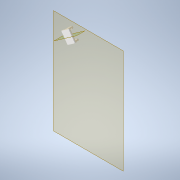
# Autodesk Inventor part: Omniscope_Camera_fix
Saved by Autodesk Inventor 2022 (Build 260153000, 153)
## iProperties
Created: 2022-05-26
Part Number: Omniscope_Camera_fix
Material: Generisch
Document SubType Name: Modeling
Designer: diederichbenedict
Density: 1 g/cm^3
Appearance: Vorgabe
Author: diederichbenedict
Autodesk Inventor part; units mm, degrees
ref_plane "YZ Plane" through (0, 0, 0) normal (1, 0, 0) x (0, 1, 0)
ref_plane "XZ Plane" through (0, 0, 0) normal (0, 1, 0) x (-1, 0, 0)
ref_plane "XY Plane" through (0, 0, 0) normal (0, 0, 1) x (1, 0, 0)
ref_plane "Arbeitsebene1" through (8.2312, -3.2392, 2) normal (0, 0, 1) x (1, 0, 0)
sketch "Skizze1" plane through (8.2312, -3.2392, 2) normal (0, 0, 1) x (1, 0, 0)
  arc A0 (-29.666, 52.3362) -> (-30.2278, 49.15) centre (-26.4114, 50.1197) ccw projected
  line L0 (-30.4697, 49.0886) -> (-31.8651, 51.0813) projected
  line L1 (-27.3731, 44.6661) -> (-28.7684, 46.6589) projected
  line L2 (-25.3803, 46.0614) -> (-27.3731, 44.6661) projected
  spline S0 degree 3 poles (-25.3803, 46.0614) (-25.4758, 46.0372) (-25.5717, 46.0164) (-25.765, 45.9815) (-25.8623, 45.9675) (-25.9823, 45.9545) (-26.0046, 45.9522) (-26.0633, 45.9468) (-26.0993, 45.944) (-26.1701, 45.9393) (-26.2048, 45.9374) (-26.2421, 45.9359) (-26.244, 45.9358) (-26.3578, 45.9313) (-26.4696, 45.9314) (-26.6928, 45.9405) (-26.8042, 45.9495) (-26.9899, 45.972) (-27.0643, 45.983) (-27.2355, 46.0132) (-27.3315, 46.0336) (-27.5218, 46.0812) (-27.6161, 46.1083) (-27.7358, 46.1473) (-27.7619, 46.1561) (-27.8204, 46.1765) (-27.8532, 46.1884) (-27.9183, 46.2129) (-27.9507, 46.2255) (-27.9876, 46.2405) (-27.9928, 46.2426) (-28.0892, 46.282) (-28.1788, 46.3225) (-28.3547, 46.4094) (-28.4411, 46.456) (-28.6083, 46.5538) (-28.6891, 46.6048) (-28.7684, 46.6589) knots 0 0 0 0 0.084049 0.084049 0.16831 0.16831 0.1875 0.1875 0.21875 0.21875 0.248427 0.248427 0.25 0.25 0.343462 0.343462 0.437098 0.437098 0.5 0.5 0.582124 0.582124 0.664424 0.664424 0.6875 0.6875 0.716281 0.716281 0.74522 0.74522 0.75 0.75 0.834095 0.834095 0.918237 0.918237 1 1 1 1 projected
  line L3 (-20.9578, 49.1581) -> (-22.9506, 47.7627) projected
  line L4 (-22.3532, 51.1509) -> (-20.9578, 49.1581) projected
  spline S1 degree 3 poles (-22.3532, 51.1509) (-22.3289, 51.0554) (-22.3081, 50.9594) (-22.2732, 50.7662) (-22.2592, 50.6689) (-22.2462, 50.5488) (-22.244, 50.5265) (-22.2385, 50.4679) (-22.2357, 50.4318) (-22.231, 50.3611) (-22.2292, 50.3263) (-22.2276, 50.289) (-22.2276, 50.2871) (-22.2231, 50.1733) (-22.2231, 50.0616) (-22.2322, 49.8384) (-22.2412, 49.727) (-22.2637, 49.5413) (-22.2747, 49.4668) (-22.3049, 49.2957) (-22.3254, 49.1997) (-22.3729, 49.0094) (-22.4, 48.915) (-22.4391, 48.7954) (-22.4479, 48.7693) (-22.4682, 48.7107) (-22.4801, 48.678) (-22.5046, 48.6128) (-22.5173, 48.5804) (-22.5322, 48.5436) (-22.5343, 48.5384) (-22.5738, 48.442) (-22.6142, 48.3524) (-22.7012, 48.1764) (-22.7477, 48.09) (-22.8455, 47.9229) (-22.8966, 47.842) (-22.9506, 47.7627) knots 0 0 0 0 0.084049 0.084049 0.16831 0.16831 0.1875 0.1875 0.21875 0.21875 0.248427 0.248427 0.25 0.25 0.343462 0.343462 0.437098 0.437098 0.5 0.5 0.582124 0.582124 0.664424 0.664424 0.6875 0.6875 0.716281 0.716281 0.74522 0.74522 0.75 0.75 0.834095 0.834095 0.918237 0.918237 1 1 1 1 projected
  line L5 (-25.4498, 55.5734) -> (-24.0545, 53.5806) projected
  line L6 (-27.4426, 54.178) -> (-25.4498, 55.5734) projected
  spline S2 degree 3 poles (-27.4426, 54.178) (-27.3471, 54.2023) (-27.2511, 54.2231) (-27.0579, 54.2579) (-26.9606, 54.272) (-26.8406, 54.285) (-26.8183, 54.2872) (-26.7596, 54.2926) (-26.7236, 54.2955) (-26.6528, 54.3001) (-26.6181, 54.302) (-26.5807, 54.3035) (-26.5789, 54.3036) (-26.4651, 54.3081) (-26.3533, 54.308) (-26.1301, 54.299) (-26.0187, 54.29) (-25.833, 54.2675) (-25.7586, 54.2564) (-25.5874, 54.2262) (-25.4914, 54.2058) (-25.3011, 54.1582) (-25.2067, 54.1311) (-25.0871, 54.0921) (-25.061, 54.0833) (-25.0025, 54.0629) (-24.9697, 54.0511) (-24.9046, 54.0266) (-24.8722, 54.0139) (-24.8353, 53.999) (-24.8301, 53.9969) (-24.7337, 53.9574) (-24.6441, 53.917) (-24.4681, 53.83) (-24.3817, 53.7835) (-24.2146, 53.6857) (-24.1337, 53.6346) (-24.0545, 53.5806) knots 0 0 0 0 0.084049 0.084049 0.16831 0.16831 0.1875 0.1875 0.21875 0.21875 0.248427 0.248427 0.25 0.25 0.343462 0.343462 0.437098 0.437098 0.5 0.5 0.582124 0.582124 0.664424 0.664424 0.6875 0.6875 0.716281 0.716281 0.74522 0.74522 0.75 0.75 0.834095 0.834095 0.918237 0.918237 1 1 1 1 projected
  line L7 (-27.0245, 40.5346) -> (-35.6282, 52.8219)
  line L8 (-35.6282, 52.8219) -> (-25.7984, 59.7048)
  line L9 (-25.7984, 59.7048) -> (-17.1947, 47.4175)
  line L10 (-17.1947, 47.4175) -> (-27.0245, 40.5346)
  line L11 (-27.0245, 40.5346) -> (-25.7984, 59.7048) construction
  line L12 (-35.6282, 52.8219) -> (-17.1947, 47.4175) construction
  line L13 (-27.0245, 40.5346) -> (-12.0245, 40.5346) construction
  circle A1 centre (-26.4114, 50.1197) radius 4.5
  circle A2 centre (-26.4114, 50.1197) radius 3.95
  point P0 (-8.2312, 3.2392)
  point P1 (-24.4756, 54.182)
  point P2 (-21.932, 50.5494)
  point P3 (-22.3491, 48.1839)
  point P4 (-25.9817, 45.6403)
  point P5 (-28.3473, 46.0574)
  point P6 (-26.8411, 54.5992)
  dimension "d0" = 125
  dimension "d1" = 15
  dimension "d2" = 12
  dimension "d3" = 9
  dimension "d16" = 7.9
  constraints: 14 end point, 2 centre point, 2 coincident, 2 midpoint, 2 parallel, 1 equal length, 1 horizontal, 1 perpendicular
  measures "d0" angle of L13 L7
  measures "d1" distance between parallel lines of L8 L10
  measures "d2" distance between parallel lines of L7 L9
  measures "d3" diameter of A1
  measures "d16" diameter of A2
extrude "Extrusion1" add sketch "Skizze1" along normal mid plane 2 contours L1 A1 L2 | A1 L6 S2 L5 L4 S1 L3 L2 S0 L1 | L1 S0 L2 A1 | A1 L4 L3 | L3 S1 L4 A1 | A1 L5 S2 L6 | L6 L5 A1 | L7 L8 L9 L10 | A2
sketch "Skizze2" plane through (-17.5671, 56.4656, 3) normal (0.819152, 0.5735764, 0) x (0, 0, -1)
  line L0 (2, 0) -> (2, -15) projected
  line L1 (2, 0) -> (0, 0) projected
  line L2 (0, -15) -> (0, 0) projected
  line L3 (0, -15) -> (2, -15) projected
  line L4 (2, 0) -> (2, -15) projected
  line L5 (2, -15) -> (8.3, -15)
  line L6 (8.3, -15) -> (8.3, -13.5)
  line L7 (8.3, -13.5) -> (6.3, -12.5)
  line L8 (6.3, -12.5) -> (6.3, -13.5)
  line L9 (6.3, -13.5) -> (2, -13.5)
  line L10 (6, -33.1362) -> (6, 10.1688) projected
  point P0 (3, -56.33)
  point P1 (2, -13.5)
  dimension "d6" = 1.5
  dimension "d7" = 0
  dimension "d8" = 1
  dimension "d9" = 0.3
  dimension "d10" = 2
  constraints: 10 end point, 2 perpendicular, 1 horizontal, 1 parallel, 1 point on line
  measures "d6" distance between parallel lines of L5 L9
  measures "d7" vertical distance of L6.end L8.end
  measures "d8" distance of L8.end L7.end
  measures "d9" distance from line of L10 L7.end
  measures "d10" distance between parallel lines of L8 L6
extrude "Extrusion2" add sketch "Skizze2" against normal up to surface (12 mm away) contours L9 L10 L5 L0 | L9 L8 L7 L6 L5 L10
chamfer "Fase1" distance 2 angle 45 1 edges at (-14.7388, 41.9656, 1)
ref_plane "Arbeitsebene2" through (-13.2653, 50.322, -5.3) normal (0.5735764, -0.819152, 0) x (0.819152, 0.5735764, 0)
mirror "Spiegeln1" about plane through (-13.2653, 50.322, -5.3) normal (0.5735764, -0.819152, 0) of "Extrusion2", "Fase1"
sketch "Skizze3" plane through (-27.3969, 49.5827, 3) normal (-0.5735764, 0.819152, 0) x (0.819152, 0.5735764, 0)
  line L0 (0, 8.3) -> (0, 0) projected
  line L1 (12, 8.3) -> (12, 0) projected
  line L2 (0, 8.3) -> (3.2, 8.3)
  line L3 (3.2, 8.3) -> (3.2, 2)
  line L4 (3.2, 2) -> (0, 2)
  line L5 (0, 2) -> (0, 8.3)
  line L6 (12, 8.3) -> (8.8, 8.3)
  line L7 (8.8, 8.3) -> (8.8, 2)
  line L8 (8.8, 2) -> (12, 2)
  line L9 (12, 2) -> (12, 8.3)
  point P0 (-5.9972, 3)
  point P1 (12, 2)
  point P2 (0, 2)
  dimension "d19" = 3.2
  dimension "d20" = 3.2
  constraints: 16 end point, 4 parallel, 2 horizontal, 2 perpendicular
  measures "d19" distance between parallel lines of L3 L0
  measures "d20" distance between parallel lines of L1 L7
extrude "Extrusion3" cut sketch "Skizze3" against normal through all
